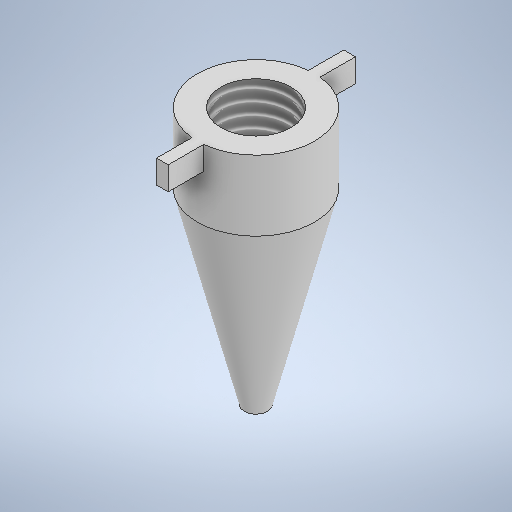
# Autodesk Inventor part: Nozzle
Saved by Autodesk Inventor 2025.2 (Build 292293000, 293)
## iProperties
Created: 2025-05-29
Part Number: Nozzle
Material: Generic
Document SubType Name: Modeling
Designer: Simon
Density: 1 g/cm^3
Appearance: Default
Author: Simon
Autodesk Inventor part; units mm, degrees
ref_plane "YZ Plane" through (0, 0, 0) normal (1, 0, 0) x (0, 1, 0)
ref_plane "XZ Plane" through (0, 0, 0) normal (0, 1, 0) x (-1, 0, 0)
ref_plane "XY Plane" through (0, 0, 0) normal (0, 0, 1) x (1, 0, 0)
sketch "Sketch1" plane through (0, 0, 0) normal (1, 0, 0) x (0, 1, 0)
  line L0 (0, 0) -> (0, 1.5)
  line L1 (0, 1.5) -> (0, 4)
  line L2 (0, 0) -> (-11, 0)
  line L3 (-11, 0) -> (-11, 0.5)
  line L4 (-11, 0.5) -> (-3, 0.5)
  line L5 (-3, 0.5) -> (-3, 1.5)
  line L6 (-3, 1.5) -> (0, 1.5)
  line L7 (-3, 1.5) -> (-3, 2.5)
  line L8 (-3, 2.5) -> (-11, 0.5)
  line L9 (-3, 2.5) -> (0, 2.5)
  line L10 (0, 4) -> (-1, 4)
  line L11 (-1, 4) -> (-1, 2.5)
  line L12 (0, 0) -> (0, -4)
  line L13 (0, -4) -> (-1, -4)
  line L14 (-1, -4) -> (-1, -1.5)
  line L15 (-1, -1.5) -> (0, -1.5)
  line L16 (-11, 0.5) -> (-11, 0.4)
  line L17 (-11, 0.4) -> (-3, 1.5)
  line L18 (-1, 2.5) -> (-1, 1.5)
  dimension "d0" = 1.5
  dimension "d1" = 2.5
  dimension "d2" = 11
  dimension "d3" = 0.5
  dimension "d4" = 8
  dimension "d5" = 1
  dimension "d6" = 1
  dimension "d7" = 1
  dimension "d8" = 4
  dimension "d9" = 1
  dimension "d10" = 2.5
  dimension "d11" = 0.1
  constraints: 38 end point, 9 point on line, 4 perpendicular, 2 horizontal, 2 parallel, 2 vertical
  measures "d0" distance of L0.start L0.end
  measures "d1" distance of L0.end L1.end
  measures "d2" distance of L0.start L2.end
  measures "d3" distance of L2.end L3.end
  measures "d4" distance of L3.end L4.end
  measures "d5" distance of L4.end L5.end
  measures "d6" distance of L5.end L7.end
  measures "d7" distance of L1.end L10.end
  measures "d8" distance of L0.start L12.end
  measures "d9" distance of L12.end L13.end
  measures "d10" distance of L13.end L14.end
  measures "d11" distance of L3.end L16.end
revolve "Revolution1" add sketch "Sketch1" angle 360 about axis through (0, 0, 0) along (0, -1, 0) contours L6 L18 L9 L1 | L6 L7 L9 L18 | L3 L4 L17 | L17 L4 L8 L7
extrude "Extrusion1" add sketch "Sketch1" along normal mid plane 0.5 contours L6 L18 L9 L1 | L9 L11 L10 L1 | L12 L13 L14 L15
thread "Thread1" size "M3x0.5" class "6H" standard "ISO Metric profile" full length
body "Solid1"
